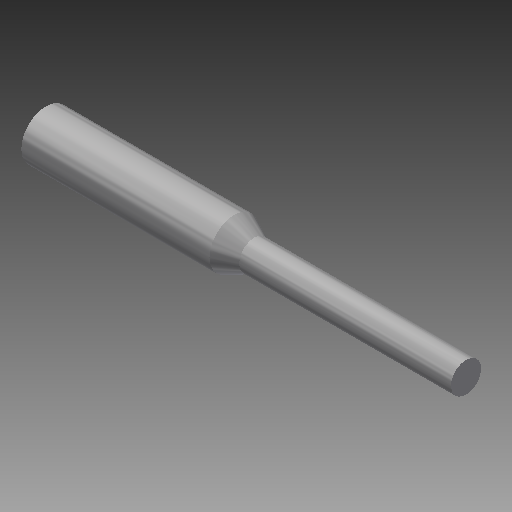
# Autodesk Inventor part: Shaft
Saved by Autodesk Inventor 2019 (Build 230136000, 136)
## iProperties
Created: 2019-07-13
Part Number: Shaft
Material: Steel
Document SubType Name: Modeling
Designer: Lino P
Density: 7.85 g/cm^3
Appearance: Steel
Mass: 325.469 g
Surface Area: 99.1849 cm^2
Volume: 41.4611 cm^3
CustomPartVersion: 1
Author: Lino P
Autodesk Inventor part; units mm, degrees
ref_plane "Start Plane" through (0, 0, 0) normal (1, 0, 0) x (0, 1, 0)
ref_plane "XZ Plane" through (0, 0, 0) normal (0, 1, 0) x (-1, 0, 0)
ref_plane "XY Plane" through (0, 0, 0) normal (0, 0, 1) x (1, 0, 0)
sketch "Main Sketch" plane through (0, 0, 0) normal (0, 0, 1) x (1, 0, 0)
  line L0 (0, 0) -> (179.1, 0)
  line L1 (0, 0) -> (0, 10.5)
  line L2 (0, 10.5) -> (80.2, 10.5)
  line L3 (80.2, 10.5) -> (88.8, 6.425)
  line L4 (179.1, 6.425) -> (179.1, 0)
  line L5 (88.8, 6.425) -> (179.1, 6.425)
  dimension "d3" = 21
  dimension "d4" = 12.85
  constraints: 12 end point, 4 horizontal, 2 vertical
  measures "d3" diameter of L2 L0
  measures "d4" diameter of L5 L0
revolve "Revolution1" add sketch "Main Sketch" angle 360 about axis through (0, 0, 0) along (1, 0, 0)
body "Solid1"
